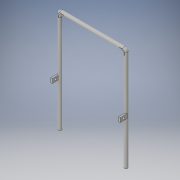
# Autodesk Inventor part: support
Saved by Autodesk Inventor 2016 (Build 200138000, 138)
## iProperties
Created: 2019-01-25
Part Number: support
Material: Generic
Document SubType Name: Modeling
Designer: Matthew Reese
Density: 1 g/cm^3
Appearance: Default
Author: Matthew Reese
Autodesk Inventor part; units mm, degrees
ref_plane "YZ Plane" through (0, 0, 0) normal (1, 0, 0) x (0, 1, 0)
ref_plane "XZ Plane" through (0, 0, 0) normal (0, 1, 0) x (-1, 0, 0)
ref_plane "XY Plane" through (0, 0, 0) normal (0, 0, 1) x (1, 0, 0)
sketch "Sketch1" plane through (0, 0, 0) normal (0, 0, 1) x (1, 0, 0)
  line L0 (-203.2, -6.35) -> (-203.2, 584.2)
  arc A0 (-184.15, 603.25) -> (-203.2, 584.2) centre (-184.15, 584.2) ccw
  line L1 (-184.15, -6.35) -> (-184.15, 565.15)
  arc A1 (-165.1, 584.2) -> (-184.15, 565.15) centre (-165.1, 565.15) ccw
  line L2 (-203.2, -6.35) -> (-184.15, -6.35)
  line L3 (203.2, -6.35) -> (203.2, 584.2)
  arc A2 (203.2, 584.2) -> (184.15, 603.25) centre (184.15, 584.2) ccw
  line L4 (184.15, -6.35) -> (184.15, 565.15)
  arc A3 (184.15, 565.15) -> (165.1, 584.2) centre (165.1, 565.15) ccw
  line L5 (203.2, -6.35) -> (184.15, -6.35)
  line L6 (165.1, 584.2) -> (-165.1, 584.2)
  line L7 (-184.15, 603.25) -> (184.15, 603.25)
  point P0 (0, 0)
  dimension "d7" = 406.4
  dimension "d31" = 609.6
  dimension "d32" = 609.6
  dimension "d33" = 19.05
  constraints: 16 end point, 8 point on circle, 4 centre point, 2 horizontal, 2 parallel, 2 tangent, 2 vertical
  measures "d7" distance of L0.end L3.end
  measures "d31" distance between parallel lines of L5 L7
  measures "d32" distance between parallel lines of L7 L2
  measures "d33" distance between parallel lines of L6 L7
extrude "Extrusion1" add sketch "Sketch1" along normal mid plane 19.05
fillet "Fillet1" radius 9.525 20 edges at (178.5704, 578.6204, 9.525) (0, 584.2, 9.525) (-178.5704, 578.6204, 9.525) (-184.15, 279.4, 9.525) (184.15, 279.4, 9.525) (197.6204, 597.6704, 9.525) (0, 603.25, 9.525) (-197.6204, 597.6704, 9.525) (-203.2, 288.925, 9.525) (203.2, 288.925, 9.525) (197.6204, 597.6704, -9.525) (0, 603.25, -9.525) (-197.6204, 597.6704, -9.525) (-203.2, 288.925, -9.525) (203.2, 288.925, -9.525) (178.5704, 578.6204, -9.525) (0, 584.2, -9.525) (-178.5704, 578.6204, -9.525) (-184.15, 279.4, -9.525) (184.15, 279.4, -9.525)
sketch "Sketch2" plane through (0, 0, 0) normal (0, 0, 1) x (1, 0, 0)
  line L0 (203.2, 584.2) -> (203.2, -6.35) projected
  line L1 (203.2, 247.65) -> (193.675, 247.65)
  line L2 (193.675, 247.65) -> (193.675, 273.05)
  line L3 (193.675, 273.05) -> (203.2, 273.05)
  line L4 (203.2, 273.05) -> (203.2, 247.65)
  line L5 (203.2, -6.35) -> (184.15, -6.35) projected
  line L6 (-203.2, -6.35) -> (-203.2, 584.2) projected
  line L7 (-203.2, 273.05) -> (-193.675, 273.05)
  line L8 (-193.675, 273.05) -> (-193.675, 247.65)
  line L9 (-193.675, 247.65) -> (-203.2, 247.65)
  line L10 (-203.2, 247.65) -> (-203.2, 273.05)
  line L11 (-184.15, -6.35) -> (-203.2, -6.35) projected
  point P0 (0, 0)
  dimension "d13" = 254
  dimension "d14" = 25.4
  dimension "d15" = 9.525
  dimension "d16" = 25.4
  dimension "d17" = 254
  dimension "d34" = 387.35
  constraints: 16 end point, 4 parallel, 2 horizontal, 2 perpendicular, 2 point on line
  measures "d13" distance between parallel lines of L5 L1
  measures "d14" distance between parallel lines of L1 L3
  measures "d15" distance of L8.end L9.end
  measures "d16" distance of L7.end L8.end
  measures "d17" distance from line of L11 L8.end
  measures "d34" distance between parallel lines of L8 L2
extrude "Extrusion2" add sketch "Sketch2" along normal blind 44.45
sketch "Sketch3" plane through (203.2, 247.65, 0) normal (1, 0, 0) x (0, 0, -1)
  line L0 (0, 25.4) -> (-44.45, 25.4) projected
  line L1 (-44.45, 0) -> (-44.45, 25.4) projected
  point P0 (0, -247.65)
  point P1 (-25.4, 12.7)
  dimension "d20" = 12.7
  dimension "d21" = 19.05
  measures "d20" distance from line of L0 point (-25.4, 12.7)
  measures "d21" distance from line of L1 point (-25.4, 12.7)
hole "Hole1" at (203.2, 260.35, 25.4) direction (-1, 0, 0) diameter 12.7 end through all
body "Solid1"
